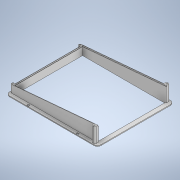
# Autodesk Inventor part: mainBody
Saved by Autodesk Inventor 2020.3 (Build 243373000, 373)
## iProperties
Created: 2021-03-06
Part Number: mainBody
Material: Generic
Document SubType Name: Modeling
Designer: allofus
Density: 1 g/cm^3
Appearance: Default
Author: allofus
Autodesk Inventor part; units mm, degrees
ref_plane "YZ Plane" through (0, 0, 0) normal (1, 0, 0) x (0, 1, 0)
ref_plane "XZ Plane" through (0, 0, 0) normal (0, 1, 0) x (-1, 0, 0)
ref_plane "XY Plane" through (0, 0, 0) normal (0, 0, 1) x (1, 0, 0)
sketch "panelconnect" plane through (0, 0, 0) normal (0, 1, 0) x (-1, 0, 0)
  circle A0 centre (0, 0) radius 2.5
  circle A1 centre (115, 0) radius 2.5
  circle A2 centre (115, 173) radius 2.5
  circle A3 centre (0, 173) radius 2.5
  line L0 (57.2025, 240.8064) -> (94.1768, 240.8064)
  line L1 (94.1768, 240.8064) -> (82.9725, 250.4701)
  line L2 (82.9725, 250.4701) -> (82.9725, 230.5824)
  line L3 (82.9725, 230.5824) -> (94.1768, 240.8064)
  line L4 (172.5, 184) -> (-57.5, 184)
  line L5 (-57.5, 184) -> (-57.5, -11)
  line L6 (-57.5, -11) -> (172.5, -11)
  line L7 (172.5, -11) -> (172.5, 184)
  line L8 (-39.5, 166) -> (154.5, 166)
  line L9 (154.5, 166) -> (154.5, 7)
  line L10 (154.5, 7) -> (-39.5, 7)
  line L11 (-39.5, 7) -> (-39.5, 166)
  line L12 (164.5, 176) -> (-49.5, 176)
  line L13 (-49.5, 176) -> (-49.5, -3)
  line L14 (-49.5, -3) -> (164.5, -3)
  line L15 (164.5, -3) -> (164.5, 176)
  dimension "d0" = 5
  dimension "d1" = 5
  dimension "d3" = 5
  dimension "d7" = 5
  dimension "d11" = 195
  dimension "d14" = 18
  dimension "d15" = 10
  dimension "d54" = 115
  dimension "d55" = 57.5
  dimension "d56" = 57.5
  dimension "d57" = 230
  dimension "d58" = 173
  dimension "d61" = 11
  dimension "d62" = 57.5
  dimension "d64" = 57.5
  dimension "d65" = 11
  constraints: 32 end point, 6 parallel, 4 centre point, 4 perpendicular, 3 horizontal, 1 coincident, 1 vertical, 6 other
  measures "d0" diameter of A0
  measures "d1" diameter of A1
  measures "d3" diameter of A2
  measures "d7" diameter of A3
  measures "d11" distance of L5.end L4.end
  measures "d14" distance between parallel lines of L4 L8
  measures "d15" distance between parallel lines of L8 L12
  measures "d54" distance of A1.centre point (0, 0)
  measures "d55" horizontal distance of A1.centre L6.end
  measures "d56" horizontal distance of L5.end point (0, 0)
  measures "d57" distance of L5.end L6.end
  measures "d58" distance of A2.centre A1.centre
  measures "d61" vertical distance of L4.end A3.centre
  measures "d62" horizontal distance of L4.end A3.centre
  measures "d64" horizontal distance of L4.start A2.centre
  measures "d65" vertical distance of L4.start A2.centre
extrude "panelExtrude" add sketch "panelconnect" along normal blind 2 contours L15 L14 L13 L12
sketch "Sketch2" plane through (0, 2, 0) normal (0, 1, 0) x (1, 0, 0)
  line L0 (39.5, -7) -> (39.5, -166) projected
  line L1 (-154.5, -166) -> (39.5, -166)
  line L2 (39.5, -166) -> (39.5, -7)
  line L3 (39.5, -7) -> (-154.5, -7)
  line L4 (-154.5, -7) -> (-154.5, -166)
  line L5 (41.5, -168) -> (-156.5, -168)
  line L6 (-156.5, -168) -> (-156.5, -5)
  line L7 (-156.5, -5) -> (41.5, -5)
  line L8 (41.5, -5) -> (41.5, -168)
  line L9 (39.5, -7) -> (64.2045, -7)
  line L10 (39.5, -166) -> (-154.5, -166) projected
  line L11 (39.5, -166) -> (69.5542, -166)
  line L12 (-156.5, -5) -> (-156.5, -168)
  line L13 (41.5, -168) -> (33.5, -168)
  line L14 (33.5, -168) -> (33.5, -174)
  line L15 (33.5, -174) -> (41.5, -174)
  line L16 (41.5, -174) -> (41.5, -168)
  line L17 (41.5, -5) -> (33.5, -5)
  line L18 (33.5, -5) -> (33.5, 1)
  line L19 (33.5, 1) -> (41.5, 1)
  line L20 (41.5, 1) -> (41.5, -5)
  circle A0 centre (37.5, -171) radius 1.55
  circle A1 centre (37.5, -2) radius 1.55
  line L21 (-156.5, -168) -> (-162.5, -168)
  line L22 (-162.5, -168) -> (-162.5, -162)
  line L23 (-162.5, -162) -> (-156.5, -162)
  line L24 (-156.5, -162) -> (-156.5, -168)
  line L25 (-156.5, -5) -> (-162.5, -5)
  line L26 (-162.5, -5) -> (-162.5, -11)
  line L27 (-162.5, -11) -> (-156.5, -11)
  line L28 (-156.5, -11) -> (-156.5, -5)
  circle A2 centre (-159.5, -165) radius 1.55
  circle A3 centre (-159.5, -8) radius 1.55
  point P0 (0, 0)
  point P1 (41.5, -166)
  point P2 (41.5, -7)
  point P3 (-156.5, -5)
  dimension "d18" = 2
  dimension "d28" = 8
  dimension "d29" = 6
  dimension "d30" = 6
  dimension "d34" = 3.1
  dimension "d35" = 3
  dimension "d36" = 4
  dimension "d37" = 3.1
  dimension "d38" = 3
  dimension "d39" = 4
  dimension "d42" = 6
  dimension "d43" = 6
  dimension "d44" = 6
  dimension "d45" = 6
  dimension "d46" = 3.1
  dimension "d47" = 3
  dimension "d48" = 3
  dimension "d49" = 3.1
  dimension "d50" = 3
  dimension "d51" = 3
  constraints: 54 end point, 12 parallel, 7 perpendicular, 6 horizontal, 4 centre point, 1 point on line, 3 other
  measures "d18" distance between parallel lines of L1 L5
  measures "d28" distance of L15.end L14.end
  measures "d29" distance of L14.end L13.end
  measures "d30" distance of L17.end L18.end
  measures "d34" diameter of A0
  measures "d35" vertical distance of L15.end A0.centre
  measures "d36" horizontal distance of A0.centre L15.end
  measures "d37" diameter of A1
  measures "d38" vertical distance of L19.end A1.centre
  measures "d39" horizontal distance of L19.end A1.centre
  measures "d42" distance of L22.end L23.end
  measures "d43" distance of L21.end L22.end
  measures "d44" distance of L27.end L26.end
  measures "d45" distance of L26.end L25.end
  measures "d46" diameter of A2
  measures "d47" horizontal distance of L23.end A2.centre
  measures "d48" horizontal distance of A2.centre L23.end
  measures "d49" diameter of A3
  measures "d50" horizontal distance of L12.start A3.centre
  measures "d51" horizontal distance of A3.centre L6.end
extrude "bodyExtrude" add sketch "Sketch2" along normal blind 35 contours L3 L4 L1 L11 L8 L5 L6 L7 L9 | L7 L18 L19 L20 | L16 L15 L14 L5 | L6 L27 L26 L25 | L21 L22 L23 L6
sketch "Sketch3" plane through (-161.5, 2, 168) normal (0, 0, 1) x (1, 0, 0)
  line L0 (203, 0) -> (203, 35) projected
  line L1 (203, 35) -> (-34.1829, 14.2492)
  line L2 (203, 35) -> (441.0889, 35) construction
  line L3 (7, 35) -> (203, 35) projected
  line L4 (-1, 0) -> (-1, 35) projected
  line L5 (-1, 17.5) -> (-1, 35)
  line L6 (203, 35) -> (195, 35) projected
  line L7 (-1, 35) -> (203, 35)
  point P0 (161.5, -2)
  point P1 (-1, 17.1523)
  dimension "d22" = 175
  constraints: 8 end point, 1 collinear, 1 equal length, 1 horizontal, 1 midpoint, 1 vertical
  measures "d22" angle of L1 L2
extrude "baseAngle" cut sketch "Sketch3" against normal mid plane 398.4625
sketch "Sketch4" plane through (-161.5, 19.2398, 168) normal (-0.0871557, 0.9961947, 0) x (0.9961947, 0.0871557, 0)
  line L0 (7.0267, 161) -> (7.0267, 2) projected
  line L1 (7.0267, 2) -> (203.6093, 2)
  line L2 (203.6093, 2) -> (203.6093, 161)
  line L3 (203.6093, 161) -> (7.0267, 161)
  line L4 (7.0267, 161) -> (7.0267, 2)
  line L5 (6.0267, 162) -> (204.6093, 162)
  line L6 (204.6093, 162) -> (204.6093, 1)
  line L7 (204.6093, 1) -> (6.0267, 1)
  line L8 (6.0267, 1) -> (6.0267, 162)
  point P0 (159.2086, 168)
  point P1 (7.0267, 21.4312)
  dimension "d25" = 1
  constraints: 16 end point, 4 parallel, 2 perpendicular, 1 horizontal, 3 other
  measures "d25" distance between parallel lines of L3 L5
extrude "bodyDetent" cut sketch "Sketch4" against normal blind 2 contours L3 L2 L1 L0 | L5 L6 L7 L8
fillet "Fillet1" radius 8.35 4 edges at (49.5, 1, -3) (-164.5, 1, -3) (-164.5, 1, 176) (49.5, 1, 176)
fillet "Fillet2" radius 3 8 edges at (33.5, 19.15, 174) (41.5, 19.5, 174) (41.5, 19.5, -1) (33.5, 19.15, -1) (-162.5, 10.5762, 11) (-162.5, 10.5762, 5) (-162.5, 10.5762, 162) (-162.5, 10.5762, 168)
body "Solid1"
